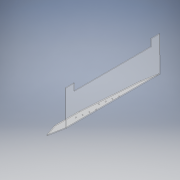
# Autodesk Inventor part: アームシールド1
Saved by Autodesk Inventor 2020 (Build 240168000, 168)
## iProperties
Created: 2019-09-16
Part Number: アームシールド1
Material: ポリカーボネート、クリア
Document SubType Name: Modeling
Designer: 雪村
Density: 1.2 g/cm^3
Appearance: ポリカーボネート - クリア
Mass: 137.865 g
Surface Area: 1168.83 cm^2
Volume: 114.888 cm^3
Author: 雪村
Autodesk Inventor part; units mm, degrees
ref_plane "YZ Plane" through (0, 0, 0) normal (1, 0, 0) x (0, 1, 0)
ref_plane "XZ Plane" through (0, 0, 0) normal (0, 1, 0) x (-1, 0, 0)
ref_plane "XY Plane" through (0, 0, 0) normal (0, 0, 1) x (1, 0, 0)
sketch "スケッチ1" plane through (0, 0, 0) normal (0, 0, 1) x (1, 0, 0)
  circle A0 centre (-149.101, -13.3308) radius 1.5 construction
  circle A1 centre (-160.5892, -1.6149) radius 1.5 construction
  circle A2 centre (-44.4492, 64.0137) radius 1.5 construction
  circle A3 centre (-64.4423, 49.0046) radius 1.5 construction
  circle A4 centre (-60.4494, 64.5064) radius 1.5 construction
  arc A5 (-40.2316, 58.3956) -> (-44.233, 71.0354) centre (-44.4492, 64.0137) ccw construction
  line L0 (-44.233, 71.0354) -> (-60.2332, 71.5281) construction
  arc A6 (-60.2332, 71.5281) -> (-64.1725, 70.4637) centre (-60.4494, 64.5064) ccw construction
  line L1 (-64.1725, 70.4637) -> (-165.9022, 6.8864) construction
  arc A7 (-165.9022, 6.8864) -> (-166.8262, -9.4635) centre (-160.5892, -1.6149) ccw construction
  line L2 (-166.8262, -9.4635) -> (-154.0782, -19.594) construction
  arc A8 (-154.0782, -19.594) -> (-144.2981, -19.7286) centre (-149.101, -13.3308) ccw construction
  line L3 (-144.2981, -19.7286) -> (-40.2316, 58.3956) construction
  circle A9 centre (-82.1645, 51.5544) radius 1.5 construction
  circle A10 centre (-141.748, 14.817) radius 1.5 construction
  circle A11 centre (-89.4637, 29.5642) radius 1.5 construction
  circle A12 centre (-117.4541, 8.5514) radius 1.5 construction
  circle A13 centre (-111.8449, 33.0052) radius 1.5 construction
  line L4 (-152.7009, -26.0367) -> (-305.9655, -141.0946)
  circle A14 centre (-149.101, -13.3308) radius 1.5 construction
  circle A15 centre (-149.101, -13.3308) radius 3 construction
  circle A16 centre (-149.101, -13.3308) radius 3 construction
  circle A17 centre (-160.5892, -1.6149) radius 9.025 construction
  circle A18 centre (-160.5892, -1.6149) radius 4.025
  line L5 (-152.7009, -26.0367) -> (-151.5741, -2.0382)
  line L6 (-64.1725, 70.4637) -> (-165.9022, 6.8864) construction
  line L7 (-144.2981, -19.7286) -> (-40.2316, 58.3956) construction
  line L8 (-305.9655, -141.0946) -> (-171.4423, -28.6314)
  line L9 (-160.5892, -1.6149) -> (-146.0204, -21.0215) construction
  line L10 (-146.0204, -21.0215) -> (-305.9655, -141.0946) construction
  circle A19 centre (-276.0256, -117.3678) radius 1
  circle A20 centre (-160.5892, -1.6149) radius 11
  line L11 (-171.4423, -28.6314) -> (-171.589, -1.6748)
  point P0 (0, 0)
  point P1 (0, 0)
  point P2 (0, 0)
  point P3 (-276.667, -116.6006)
  point P4 (-275.4252, -118.1676)
  point P5 (-151.8691, -8.3201)
  dimension "d6" = 22
  dimension "d0" = 6
  dimension "d1" = 8.05
  dimension "d2" = 5
  dimension "d3" = 3
  dimension "d4" = 200
  dimension "d5" = 2
  dimension "d7" = 3
  dimension "d8" = 6
  constraints: 24 end point, 19 centre point, 8 point on circle, 4 tangent, 3 coincident, 2 collinear, 2 concentric, 1 perpendicular, 42 other
  measures "d0" diameter of A15
  measures "d1" diameter of A18
  measures "d3" angle of L4 L8
  measures "d4" distance of L9.end L4.end
  measures "d5" diameter of A19
  measures "d7" angle of L5 L11
  measures "d8" diameter of A16
sketch "スケッチ2" plane through (0, 0, 0) normal (0, 0, 1) x (1, 0, 0)
  line L0 (-305.9655, -141.0946) -> (-171.4423, -28.6314) projected
  line L1 (-171.4423, -28.6314) -> (-171.589, -1.6748) projected
  line L2 (-302.5902, -138.2728) -> (-303.873, -136.7384)
  line L3 (-303.873, -136.7384) -> (-173.4475, -27.7009)
  line L4 (-173.4475, -27.7009) -> (-173.9864, 71.3562)
  line L5 (-173.9864, 71.3562) -> (-171.9864, 71.3671)
  line L6 (-171.9864, 71.3671) -> (-171.589, -1.6748)
  point P0 (0, 0)
  dimension "d9" = 2
  dimension "d10" = 2
  dimension "d11" = 100
  dimension "d14" = 170
  constraints: 10 end point, 2 parallel, 2 perpendicular, 1 collinear, 1 point on line
  measures "d9" distance of L2.start L2.end
  measures "d10" horizontal distance of L4.end L5.end
  measures "d11" distance of L5.end L0.end
  measures "d14" distance of L2.end L3.end
extrude "押し出し1" add sketch "スケッチ2" along normal blind 270
sketch "スケッチ3" plane through (0, 0, 270) normal (0, 0, 1) x (1, 0, 0)
  arc A0 (-225.7, -73.9915) -> (-224.5724, -73.0489) centre (-225.6172, -72.9448) ccw
  line L0 (-225.7, -73.9915) -> (-243.7526, -89.0838)
  arc A1 (-244.8802, -90.0264) -> (-243.7526, -89.0838) centre (-244.7975, -88.9797) ccw
  line L1 (-244.8802, -90.0264) -> (-276.667, -116.6006)
  arc A2 (-276.667, -116.6006) -> (-275.4252, -118.1676) centre (-276.0256, -117.3678) ccw
  line L2 (-275.4252, -118.1676) -> (-152.7009, -26.0367)
  line L3 (-152.7009, -26.0367) -> (-151.8691, -8.3201)
  arc A3 (-151.8691, -8.3201) -> (-171.589, -1.6748) centre (-160.5892, -1.6149) ccw
  line L4 (-171.589, -1.6748) -> (-171.4423, -28.6314)
  line L5 (-171.4423, -28.6314) -> (-186.2119, -40.979)
  arc A4 (-187.3395, -41.9217) -> (-186.2119, -40.979) centre (-187.2568, -40.8749) ccw
  line L6 (-187.3395, -41.9217) -> (-205.3922, -57.0139)
  arc A5 (-206.5197, -57.9566) -> (-205.3922, -57.0139) centre (-206.437, -56.9099) ccw
  line L7 (-206.5197, -57.9566) -> (-224.5724, -73.0489)
  circle A6 centre (-171.2358, -34.3242) radius 1.5
  circle A7 centre (-160.5892, -1.6149) radius 4.025
  point P0 (0, 0)
  point P1 (0, 0)
  constraints: 16 end point, 12 point on circle, 8 centre point, 38 other
sketch "スケッチ4" plane through (-303.873, -136.7384, 270) normal (-0.6413971, 0.7672091, 0) x (0.7672091, 0.6413971, 0)
  line L0 (234.6628, 270) -> (234.6628, 0) projected
  circle A0 centre (150.9556, 102) radius 1.5
  circle A1 centre (125.9556, 102) radius 1.5
  circle A2 centre (100.9556, 102) radius 1.5
  circle A3 centre (75.9556, 102) radius 1.5
  line L1 (234.6628, 135) -> (-10.981, 135)
  circle A4 centre (150.9556, 168) radius 1.5
  circle A5 centre (125.9556, 168) radius 1.5
  circle A6 centre (100.9556, 168) radius 1.5
  circle A7 centre (75.9556, 168) radius 1.5
  line L2 (154.7693, 165) -> (132.5454, 165)
  line L3 (157.7493, 105) -> (143.6573, 105)
  point P0 (320.8377, 270)
  point P1 (150.9556, 0)
  point P2 (125.9556, 0)
  point P3 (100.9556, 0)
  point P4 (75.9556, 0)
  dimension "d15" = 3
  dimension "d16" = 3
  dimension "d17" = 3
  dimension "d18" = 3
  dimension "d20" = 33
  dimension "d27" = 3
  dimension "d28" = 3
  dimension "d29" = 60
  constraints: 8 centre point, 6 end point, 4 symmetric about line, 4 vertical alignment, 3 horizontal, 3 horizontal alignment, 1 midpoint, 4 other
  measures "d15" diameter of A0
  measures "d16" diameter of A1
  measures "d17" diameter of A2
  measures "d18" diameter of A3
  measures "d20" distance from line of A0.centre L1
  measures "d27" distance from line of A4.centre L2
  measures "d28" distance from line of A0.centre L3
  measures "d29" distance between parallel lines of L3 L2
extrude "押し出し2" cut sketch "スケッチ4" against normal through all
chamfer "面取り1" distance 100 angle 45 2 edges at (-303.2316, -137.5056, 0) (-303.2316, -137.5056, 270)
sketch "スケッチ5" plane through (-171.9864, 71.3671, 270) normal (0.9999852, 0.0054408, 0) x (0, 0, -1)
  line L0 (270, 0) -> (0, 0) projected
  line L1 (0, 0) -> (0, -99.0586) projected
  line L2 (0, 0) -> (25, 0)
  line L3 (270, 0) -> (245, 0)
  line L4 (245, 0) -> (245, -20)
  line L5 (245, -20) -> (25, -20)
  line L6 (25, -20) -> (25, 0)
  point P0 (270, -72.3018)
  dimension "d30" = 25
  dimension "d31" = 25
  dimension "d32" = 20
  constraints: 10 end point, 2 point on line, 2 vertical, 1 horizontal
  measures "d30" distance of L0.end L2.end
  measures "d31" distance of L0.start L3.end
  measures "d32" distance of L3.end L4.end
extrude "押し出し3" cut sketch "スケッチ5" against normal through all
equation "\"d8\" = d0"
